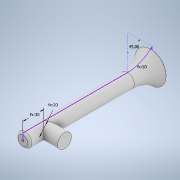
# Autodesk Inventor part: fiberHolder2
Saved by Autodesk Inventor 2022.2 (Build 262287000, 287)
## iProperties
Created: 2021-12-20
Part Number: fiberHolder2
Material: Generic
Document SubType Name: Sheet Metal
Designer: Andrei
Density: 1 g/cm^3
Appearance: Default
Sheet Metal Rule: Default
Author: Andrei
Autodesk Inventor part; units mm, degrees
ref_plane "YZ Plane" through (0, 0, 0) normal (1, 0, 0) x (0, 1, 0)
ref_plane "XZ Plane" through (0, 0, 0) normal (0, 1, 0) x (-1, 0, 0)
ref_plane "XY Plane" through (0, 0, 0) normal (0, 0, 1) x (1, 0, 0)
sketch "Sketch1" plane through (0, 0, 0) normal (1, 0, 0) x (0, 1, 0)
  line L0 (10, 0) -> (10, 150.8357)
  arc A0 (10, 0) -> (24.6447, -35.3553) centre (60, 0) ccw
  line L1 (10, 0) -> (60, 0) construction
  line L2 (24.6447, -35.3553) -> (60, 0) construction
  line L3 (24.6447, -35.3553) -> (0, -35.3553)
  line L4 (10, 150.8357) -> (0, 150.8357)
  line L5 (0, 150.8357) -> (0, -35.3553)
  circle A1 centre (0, 120.8357) radius 10
  point P0 (0, 0)
  dimension "d5" = 50
  dimension "d6" = 45
  dimension "d21" = 20
  dimension "d22" = 30
  constraints: 12 end point, 2 centre point, 2 point on circle, 1 horizontal, 1 point on line, 1 tangent, 1 vertical
  measures "d5" radius of A0
  measures "d6" angle of L1 L2
  measures "d21" diameter of A1
  measures "d22" distance from line of A1.centre L4
revolve "Revolution1" add sketch "Sketch1" angle 360 about axis through (0, 0, 150.8357) along (0, 0, -1) picked at (3.0032, 122.282) contours A0 L3 L5 A1 L0 | A1 L5 L4 L0 | A1 L5
fillet "Fillet1" radius 3 1 edges at (0, -10, 150.8357)
sketch "Sketch2" plane through (0, 0, 150.8357) normal (0, 0, 1) x (1, 0, 0)
  point P0 (0, 0)
  point P1 (0, 0)
  constraints: 1 coincident
hole "Hole1" at (0, 0, 150.8357) direction (0, 0, -1) diameter 3 end through all
fillet "Fillet2" radius 50 1 edges at (0, 1.5, -35.3553)
chamfer "Chamfer1" distance 3 angle 45 2 edges at (-24.6447, 0, -35.3553) (24.6447, 0, -35.3553)
ref_plane "Work Plane2" through (0, 10, 0) normal (-1, 0, 0) x (0, 0, 1)
ref_plane "Work Plane1" through (0, 10, 150.8357) normal (0, 1, 0) x (-1, 0, 0)
extrude "Extrusion1" add sketch "Sketch1" along normal blind 30 contours A1 L5 | L5 A1
sketch "Sketch3" plane through (0, 0, 150.8357) normal (0, 0, 1) x (1, 0, 0)
  point P0 (0, 0)
  point P1 (0, 0)
  constraints: 1 coincident
hole "Hole2" at (0, 0, 150.8357) direction (0, 0, -1) diameter 3 end through all
equation "\"d5\" = Rbend"
equation "\"d21\" = mainDiameter"
equation "\"d22\" = magnetPosition"
equation "\"d23\" = magnetPosition"
equation "\"d30\" = Thickness"
equation "\"mainDiameter\" = 20"
equation "\"channelDiameter\" = 1"
equation "\"Rbend\" = 50"
equation "\"BendRadius\" = Thickness"
equation "\"BendReliefWidth\" = Thickness"
equation "\"BendReliefDepth\" = 0.5 * Thickness"
equation "\"CornerReliefSize\" = 4 * Thickness"
equation "\"MinimumRemnant\" = 2 * Thickness"
equation "\"TransitionRadius\" = BendRadius"
equation "\"JacobiRadiusSize\" = BendRadius"
equation "\"GapSize\" = Thickness"
equation "\"magnetPosition\" = 30"
equation "\"Thickness\" = 3.048"
body "Solid1"
